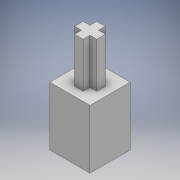
# Autodesk Inventor part: ClutchAdapter
Saved by Autodesk Inventor 2017 (Build 210142000, 142)
## iProperties
Created: 2017-02-07
Part Number: ClutchAdapter
Material: Generic
Document SubType Name: Modeling
Designer: aribu
Density: 1 g/cm^3
Appearance: Default
Author: aribu
Autodesk Inventor part; units mm, degrees
ref_plane "YZ Plane" through (0, 0, 0) normal (1, 0, 0) x (0, 1, 0)
ref_plane "XZ Plane" through (0, 0, 0) normal (0, 1, 0) x (-1, 0, 0)
ref_plane "XY Plane" through (0, 0, 0) normal (0, 0, 1) x (1, 0, 0)
sketch "Sketch1" plane through (0, 0, 0) normal (0, 0, 1) x (1, 0, 0)
  line L0 (-3.8602, 4.8039) -> (5.0398, 4.8039)
  line L1 (5.0398, 4.8039) -> (5.0398, -4.0961)
  line L2 (5.0398, -4.0961) -> (-3.8602, -4.0961)
  line L3 (-3.8602, -4.0961) -> (-3.8602, 4.8039)
  point P0 (0, 0)
  dimension "d0" = 8.9
  dimension "d1" = 8.9
  constraints: 8 end point, 2 parallel, 1 horizontal, 1 perpendicular
  measures "d0" distance of L1.end L2.end
  measures "d1" distance of L0.end L1.end
extrude "Extrusion1" add sketch "Sketch1" along normal blind 13
sketch "Sketch2" plane through (0, 0, 13) normal (0, 0, 1) x (1, 0, 0)
  line L0 (-0.3102, 2.7539) -> (1.5898, 2.7539)
  line L1 (1.5898, -2.1461) -> (-0.3102, -2.1461)
  line L2 (3.0898, 1.2539) -> (3.0898, -0.6461)
  line L3 (-1.8102, -0.6461) -> (-1.8102, 1.2539)
  line L4 (-3.8602, 4.8039) -> (5.0398, 4.8039) projected
  line L5 (-3.8602, -4.0961) -> (-3.8602, 4.8039) projected
  line L6 (5.0398, 4.8039) -> (5.0398, -4.0961) projected
  line L7 (-3.8602, -4.0961) -> (5.0398, -4.0961) projected
  line L8 (-1.8102, 1.2539) -> (-0.3102, 1.2539)
  line L9 (1.5898, 1.2539) -> (3.0898, 1.2539)
  line L10 (-0.3102, -2.1461) -> (-0.3102, -0.6461)
  line L11 (-0.3102, 1.2539) -> (-0.3102, 2.7539)
  line L12 (3.0898, -0.6461) -> (1.5898, -0.6461)
  line L13 (-0.3102, -0.6461) -> (-1.8102, -0.6461)
  line L14 (1.5898, 2.7539) -> (1.5898, 1.2539)
  line L15 (1.5898, -0.6461) -> (1.5898, -2.1461)
  point P0 (0, 0)
  dimension "d4" = 1.9
  dimension "d5" = 1.9
  dimension "d6" = 4.9
  dimension "d7" = 4.9
  constraints: 24 end point, 10 parallel, 4 perpendicular, 3 horizontal
  measures "d4" distance of L0.start L0.end
  measures "d5" distance of L2.start L2.end
  measures "d6" distance of L1.end L0.start
  measures "d7" distance of L3.end L2.start
extrude "Extrusion2" add sketch "Sketch2" along normal blind 10 contours L0 L14 L9 L2 L12 L15 L1 L10 L13 L3 L8 L11
body "Solid1"
